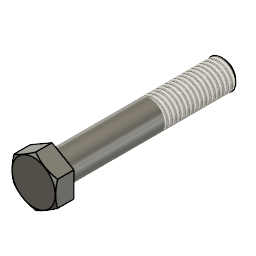
lazy boy (Autodesk Fusion 360 archive; units mm, degrees)
design "Hexagon Head Bolt ISO 4016 - M12 x 70 Steel 4.6 Plain"
description: Hexagon Head Bolt ISO 4016 - M12 x 70
part number: ISO 4016 - M12 x 70 Steel 4.6 Plain
Autodesk Fusion 360 part; units mm, degrees
sketch "Sketch1" plane through (0, 0, 0) normal (0, 1, 0) x (1, 0, 0)
  line L0 (-6, 0) -> (-6, 70)
  line L1 (-6, 70) -> (0, 70)
  line L2 (0, 70) -> (0, -7.5)
  line L3 (-6, 0) -> (-10.2852, 0)
  line L4 (-10.2852, 0) -> (-10.2852, -6.6541)
  line L5 (-8.82, -7.5) -> (0, -7.5)
  line L6 (-10.2852, -6.6541) -> (-8.82, -7.5)
  dimension "d81" = 20.5704
  dimension "d135" = 12
  dimension "d139" = 7.5
  dimension "d140" = 70
  dimension "d156" = 17.64
  dimension "d158" = 30
  constraint perpendicular L0 L1
  constraint collinear origin L1.end L2.end
  constraint perpendicular L0 L3
  constraint coincident origin L3
  constraint vertical L2
  constraint coincident L2 L5.end
  constraint coincident L0.start L3.start
  constraint coincident L0.end L1.start
  constraint vertical L4
  measures "d139" distance of L3 L5
  measures "d140" distance of L1 L3
  measures "d158" angle of L5 L6
revolve "Revolve1" add sketch "Sketch1" angle 360 about axis through (0, 0, -70) along (0, 0, 1)
sketch "Sketch8" plane through (0, 0, 7.5) normal (0, 0, 1) x (1, 0, 0)
  circle A0 centre (0, 0) radius 10.2852
  line L0 (-8.9072, -5.1426) -> (0, -10.2852)
  line L1 (0, -10.2852) -> (8.9072, -5.1426)
  line L2 (8.9072, -5.1426) -> (8.9072, 5.1426)
  line L3 (8.9072, 5.1426) -> (0, 10.2852)
  line L4 (0, 10.2852) -> (-8.9072, 5.1426)
  line L5 (-8.9072, 5.1426) -> (-8.9072, -5.1426)
  constraint coincident A0 L0.start
  constraint coincident A0.centre origin
  constraint vertical L5
extrude "Extrude5" cut sketch "Sketch8" against normal blind 7.5 contours A0 L2 | A0 L3 | A0 L1 | A0 L4 | A0 L0 | A0 L5
fillet "Fillet7" radius 0.6 1 edges at (-5.594, 2.1697, 0)
thread "Thread4" "ISO Metric profile 12.0 M12x1.75 M12x1.75 6g" major diameter 11.8335 minor diameter 9.8365 pitch 1.75 angle 60 resizes the face on face at (-5.9702, 0.5974, -46.8667) from (0, 0, -40) to (0, 0, -70)
sketch "Sketch13" plane through (0, 0, 0) normal (0, 1, 0) x (1, 0, 0)
  line L0 (0, 70) -> (0, -7.5) construction
  line L1 (0, 70) -> (-6.12, 70)
  line L2 (-6.12, 70) -> (-6.12, 68.8)
  line L3 (-6.12, 68.8) -> (-4.8, 70)
  dimension "d160" = 1.2
  dimension "d161" = 4.8
  dimension "d162" = 6.12
  constraint coincident L0.start L1.start
  constraint perpendicular L0 L1
  constraint perpendicular L1 L2
  constraint coincident L1 L3.end
  measures "d160" distance of L1 L2.end
  measures "d161" distance of L0 L3.end
  measures "d162" distance of L0.start L2
revolve "Revolve4" cut sketch "Sketch13" angle 360 about axis through (0, 0, 1.75) along (0, 0, 1)
equation "adsk_nomlen = 70.00 mm"
equation "adsk_headh = 7.50 mm"
equation "adsk_headdia = 20.5704 mm"
equation "adsk_nomdia = 12.00 mm"
equation "d81 = adsk_headdia"
equation "d89 = -adsk_headh"
equation "adsk_waflat = 18.00 mm"
equation "adsk_thrlen = 30.00 mm"
equation "adsk_midfillet = 0.60 mm"
equation "d135 = adsk_nomdia"
equation "d139 = adsk_headh"
equation "d140 = adsk_nomlen"
equation "d142 = adsk_midfillet"
equation "adsk_endpointdia = adsk_nomdia - adsk_startlen * 2"
equation "adsk_startlen = 0.1 * adsk_nomdia"
equation "d156 = adsk_waflat * 0.98"
equation "d158 = adsk_chamang2"
equation "adsk_chamang2 = 30.00 deg"
equation "d160 = adsk_startlen"
equation "d161 = adsk_endpointdia / 2"
equation "d162 = adsk_nomdia * 0.51"
equation "d166 = min(adsk_thrlen; adsk_nomlen - adsk_midfillet - 0.001 mm)"

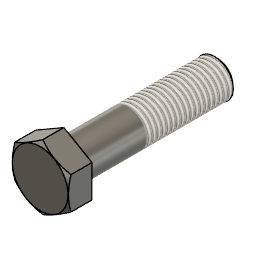
design "Hexagon Head Bolt ISO 4016 - M16 x 65 Steel 4.6 Plain"
description: Hexagon Head Bolt ISO 4016 - M16 x 65
part number: ISO 4016 - M16 x 65 Steel 4.6 Plain
Autodesk Fusion 360 part; units mm, degrees
sketch "Sketch1" plane through (0, 0, 0) normal (0, 1, 0) x (1, 0, 0)
  line L0 (-8, 0) -> (-8, 65)
  line L1 (-8, 65) -> (0, 65)
  line L2 (0, 65) -> (0, -10)
  line L3 (-8, 0) -> (-13.7136, 0)
  line L4 (-13.7136, 0) -> (-13.7136, -8.8721)
  line L5 (-11.76, -10) -> (0, -10)
  line L6 (-13.7136, -8.8721) -> (-11.76, -10)
  dimension "d81" = 27.4272
  dimension "d135" = 16
  dimension "d139" = 10
  dimension "d140" = 65
  dimension "d156" = 23.52
  dimension "d158" = 30
  constraint perpendicular L0 L1
  constraint collinear origin L1.end L2.end
  constraint perpendicular L0 L3
  constraint coincident origin L3
  constraint vertical L2
  constraint coincident L2 L5.end
  constraint coincident L0.start L3.start
  constraint coincident L0.end L1.start
  constraint vertical L4
  measures "d139" distance of L3 L5
  measures "d140" distance of L1 L3
  measures "d158" angle of L5 L6
revolve "Revolve1" add sketch "Sketch1" angle 360 about axis through (0, 0, -65) along (0, 0, 1)
sketch "Sketch8" plane through (0, 0, 10) normal (0, 0, 1) x (1, 0, 0)
  circle A0 centre (0, 0) radius 13.7136
  line L0 (-11.8763, -6.8568) -> (0, -13.7136)
  line L1 (0, -13.7136) -> (11.8763, -6.8568)
  line L2 (11.8763, -6.8568) -> (11.8763, 6.8568)
  line L3 (11.8763, 6.8568) -> (0, 13.7136)
  line L4 (0, 13.7136) -> (-11.8763, 6.8568)
  line L5 (-11.8763, 6.8568) -> (-11.8763, -6.8568)
  constraint coincident A0 L0.start
  constraint coincident A0.centre origin
  constraint vertical L5
extrude "Extrude5" cut sketch "Sketch8" against normal blind 10 contours A0 L2 | A0 L3 | A0 L1 | A0 L4 | A0 L0 | A0 L5
fillet "Fillet7" radius 0.6 1 edges at (-7.4586, 2.8929, 0)
thread "Thread4" "ISO Metric profile 16.0 M16x2 M16x2 6g" major diameter 15.822 minor diameter 13.534 pitch 2 angle 60 resizes the face on face at (-7.9602, 0.7965, -43.5333) from (0, 0, -27) to (0, 0, -65)
sketch "Sketch13" plane through (0, 0, 0) normal (0, 1, 0) x (1, 0, 0)
  line L0 (0, 65) -> (0, -10) construction
  line L1 (0, 65) -> (-8.16, 65)
  line L2 (-8.16, 65) -> (-8.16, 63.4)
  line L3 (-8.16, 63.4) -> (-6.4, 65)
  dimension "d160" = 1.6
  dimension "d161" = 6.4
  dimension "d162" = 8.16
  constraint coincident L0.start L1.start
  constraint perpendicular L0 L1
  constraint perpendicular L1 L2
  constraint coincident L1 L3.end
  measures "d160" distance of L1 L2.end
  measures "d161" distance of L0 L3.end
  measures "d162" distance of L0.start L2
revolve "Revolve4" cut sketch "Sketch13" angle 360 about axis through (0, 0, 1.75) along (0, 0, 1)
equation "adsk_nomlen = 65.00 mm"
equation "adsk_headh = 10.00 mm"
equation "adsk_headdia = 27.4272 mm"
equation "adsk_nomdia = 16.00 mm"
equation "d81 = adsk_headdia"
equation "d89 = -adsk_headh"
equation "adsk_waflat = 24.00 mm"
equation "adsk_thrlen = 38.00 mm"
equation "adsk_midfillet = 0.60 mm"
equation "d135 = adsk_nomdia"
equation "d139 = adsk_headh"
equation "d140 = adsk_nomlen"
equation "d142 = adsk_midfillet"
equation "adsk_endpointdia = adsk_nomdia - adsk_startlen * 2"
equation "adsk_startlen = 0.1 * adsk_nomdia"
equation "d156 = adsk_waflat * 0.98"
equation "d158 = adsk_chamang2"
equation "adsk_chamang2 = 30.00 deg"
equation "d160 = adsk_startlen"
equation "d161 = adsk_endpointdia / 2"
equation "d162 = adsk_nomdia * 0.51"
equation "d166 = min(adsk_thrlen; adsk_nomlen - adsk_midfillet - 0.001 mm)"
